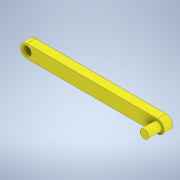
# Autodesk Inventor part: innerLink
Saved by Autodesk Inventor 2022 (Build 260153000, 153)
## iProperties
Created: 2021-12-27
Part Number: innerLink
Material: Stainless Steel
Document SubType Name: Modeling
Designer: G S SHOURIE
Density: 8 g/cm^3
Appearance: Canary
Author: G S SHOURIE
Autodesk Inventor part; units mm, degrees
ref_plane "YZ Plane" through (0, 0, 0) normal (1, 0, 0) x (0, 1, 0)
ref_plane "XZ Plane" through (0, 0, 0) normal (0, 1, 0) x (-1, 0, 0)
ref_plane "XY Plane" through (0, 0, 0) normal (0, 0, 1) x (1, 0, 0)
sketch "Sketch1" plane through (0, 0, 0) normal (0, 0, 1) x (1, 0, 0)
  line L0 (-110.5069, 7.5) -> (39.4931, 7.5)
  line L1 (39.4931, 7.5) -> (39.4931, -7.5)
  line L2 (39.4931, -7.5) -> (-110.5069, -7.5)
  line L3 (-110.5069, -7.5) -> (-110.5069, 7.5)
  arc A0 (-110.5069, 7.5) -> (-110.5069, -7.5) centre (-110.5069, 0) ccw
  arc A1 (39.4931, -7.5) -> (39.4931, 7.5) centre (39.4931, 0) ccw
  circle A2 centre (-110.5069, 0) radius 5
  point P0 (0, 0)
  dimension "d0" = 150
  dimension "d1" = 15
  dimension "d2" = 7.5
  dimension "d3" = 10
  constraints: 8 end point, 4 point on circle, 3 centre point, 2 midpoint, 2 parallel, 1 coincident, 1 horizontal, 1 perpendicular
  measures "d0" distance of L1.end L2.end
  measures "d1" distance of L0.end L1.end
  measures "d2" distance from line of L0 point (0, 0)
  measures "d3" diameter of A2
extrude "Extrusion1" add sketch "Sketch1" along normal blind 10 contours L0 L1 L2 L3 A2 | L3 A2 A0 | A1 L1
sketch "Sketch2" plane through (0, 0, 10) normal (0, 0, 1) x (1, 0, 0)
  arc A0 (39.4931, -7.5) -> (39.4931, 7.5) centre (39.4931, 0) ccw projected
  circle A1 centre (39.4931, 0) radius 5
  point P0 (0, 0)
  dimension "d6" = 10
  constraints: 1 centre point, 1 coincident
  measures "d6" diameter of A1
extrude "Extrusion2" add sketch "Sketch2" along normal blind 15
body "Solid1"
